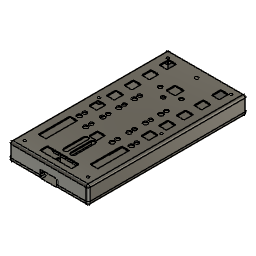
traktorino case v13 (Autodesk Fusion 360 design; units mm, degrees)
Autodesk Fusion 360 part; units mm, degrees
(part 1 of 2)
sketch "Sketch4" plane through (0, 0, 0) normal (0, 0, 1) x (1, 0, 0)
  line L0 (6.0259, 3.0477) -> (114.9323, 3.0477)
  arc A0 (114.9323, 3.0477) -> (119.7795, -1.7995) centre (114.9323, -1.7995) cw
  line L1 (119.7795, -1.7995) -> (119.7795, -228.5675)
  arc A1 (119.7795, -228.5675) -> (114.9323, -233.4147) centre (114.9323, -228.5675) cw
  line L2 (114.9323, -233.4147) -> (6.0259, -233.4147)
  arc A2 (6.0259, -233.4147) -> (1.1787, -228.5675) centre (6.0259, -228.5675) cw
  line L3 (1.1787, -228.5675) -> (1.1787, -1.7995)
  arc A3 (1.1787, -1.7995) -> (6.0259, 3.0477) centre (6.0259, -1.7995) cw
  line L4 (54.6466, -37.8457) -> (66.6101, -37.8457)
  arc A4 (66.6101, -37.8457) -> (67.4219, -38.6575) centre (66.6101, -38.6575) cw
  line L5 (67.4219, -38.6575) -> (67.4219, -51.7349)
  arc A5 (67.4219, -51.7349) -> (66.6101, -52.5468) centre (66.6101, -51.7349) cw
  line L6 (66.6101, -52.5468) -> (54.6466, -52.5468)
  arc A6 (54.6466, -52.5468) -> (53.8348, -51.7349) centre (54.6466, -51.7349) cw
  line L7 (53.8348, -51.7349) -> (53.8348, -38.6575)
  arc A7 (53.8348, -38.6575) -> (54.6466, -37.8457) centre (54.6466, -38.6575) cw
  line L8 (94.2203, -37.1462) -> (104.2753, -37.1462)
  arc A8 (104.2753, -37.1462) -> (105.0525, -37.9233) centre (104.2753, -37.9233) cw
  line L9 (105.0525, -37.9233) -> (105.0525, -50.1841)
  arc A9 (105.0525, -50.1841) -> (104.2753, -50.9613) centre (104.2753, -50.1841) cw
  line L10 (104.2753, -50.9613) -> (94.2203, -50.9613)
  arc A10 (94.2203, -50.9613) -> (93.4431, -50.1841) centre (94.2203, -50.1841) cw
  line L11 (93.4431, -50.1841) -> (93.4431, -37.9233)
  arc A11 (93.4431, -37.9233) -> (94.2203, -37.1462) centre (94.2203, -37.9233) cw
  line L12 (94.2203, -63.1605) -> (104.2753, -63.1605)
  arc A12 (104.2753, -63.1605) -> (105.0525, -63.9377) centre (104.2753, -63.9377) cw
  line L13 (105.0525, -63.9377) -> (105.0525, -76.1984)
  arc A13 (105.0525, -76.1984) -> (104.2753, -76.9756) centre (104.2753, -76.1984) cw
  line L14 (104.2753, -76.9756) -> (94.2203, -76.9756)
  arc A14 (94.2203, -76.9756) -> (93.4431, -76.1984) centre (94.2203, -76.1984) cw
  line L15 (93.4431, -76.1984) -> (93.4431, -63.9377)
  arc A15 (93.4431, -63.9377) -> (94.2203, -63.1605) centre (94.2203, -63.9377) cw
  line L16 (94.2203, -89.1736) -> (104.2753, -89.1736)
  arc A16 (104.2753, -89.1736) -> (105.0525, -89.9507) centre (104.2753, -89.9507) cw
  line L17 (105.0525, -89.9507) -> (105.0525, -102.2115)
  arc A17 (105.0525, -102.2115) -> (104.2753, -102.9887) centre (104.2753, -102.2115) cw
  line L18 (104.2753, -102.9887) -> (94.2203, -102.9887)
  arc A18 (94.2203, -102.9887) -> (93.4431, -102.2115) centre (94.2203, -102.2115) cw
  line L19 (93.4431, -102.2115) -> (93.4431, -89.9507)
  arc A19 (93.4431, -89.9507) -> (94.2203, -89.1736) centre (94.2203, -89.9507) cw
  line L20 (17.1824, -63.1605) -> (27.2374, -63.1605)
  arc A20 (27.2374, -63.1605) -> (28.0146, -63.9377) centre (27.2374, -63.9377) cw
  line L21 (28.0146, -63.9377) -> (28.0146, -76.1984)
  arc A21 (28.0146, -76.1984) -> (27.2374, -76.9756) centre (27.2374, -76.1984) cw
  line L22 (27.2374, -76.9756) -> (17.1824, -76.9756)
  arc A22 (17.1824, -76.9756) -> (16.4052, -76.1984) centre (17.1824, -76.1984) cw
  line L23 (16.4052, -76.1984) -> (16.4052, -63.9377)
  arc A23 (16.4052, -63.9377) -> (17.1824, -63.1605) centre (17.1824, -63.9377) cw
  line L24 (17.1824, -89.1736) -> (27.2374, -89.1736)
  arc A24 (27.2374, -89.1736) -> (28.0146, -89.9507) centre (27.2374, -89.9507) cw
  line L25 (28.0146, -89.9507) -> (28.0146, -102.2115)
  arc A25 (28.0146, -102.2115) -> (27.2374, -102.9887) centre (27.2374, -102.2115) cw
  line L26 (27.2374, -102.9887) -> (17.1824, -102.9887)
  arc A26 (17.1824, -102.9887) -> (16.4052, -102.2115) centre (17.1824, -102.2115) cw
  line L27 (16.4052, -102.2115) -> (16.4052, -89.9507)
  arc A27 (16.4052, -89.9507) -> (17.1824, -89.1736) centre (17.1824, -89.9507) cw
  line L28 (17.1824, -115.1879) -> (27.2374, -115.1879)
  arc A28 (27.2374, -115.1879) -> (28.0146, -115.965) centre (27.2374, -115.965) cw
  line L29 (28.0146, -115.965) -> (28.0146, -128.2258)
  arc A29 (28.0146, -128.2258) -> (27.2374, -129.003) centre (27.2374, -128.2258) cw
  line L30 (27.2374, -129.003) -> (17.1824, -129.003)
  arc A30 (17.1824, -129.003) -> (16.4052, -128.2258) centre (17.1824, -128.2258) cw
  line L31 (16.4052, -128.2258) -> (16.4052, -115.965)
  arc A31 (16.4052, -115.965) -> (17.1824, -115.1879) centre (17.1824, -115.965) cw
  line L32 (94.2203, -115.1879) -> (104.2753, -115.1879)
  arc A32 (104.2753, -115.1879) -> (105.0525, -115.965) centre (104.2753, -115.965) cw
  line L33 (105.0525, -115.965) -> (105.0525, -128.2258)
  arc A33 (105.0525, -128.2258) -> (104.2753, -129.003) centre (104.2753, -128.2258) cw
  line L34 (104.2753, -129.003) -> (94.2203, -129.003)
  arc A34 (94.2203, -129.003) -> (93.4431, -128.2258) centre (94.2203, -128.2258) cw
  line L35 (93.4431, -128.2258) -> (93.4431, -115.965)
  arc A35 (93.4431, -115.965) -> (94.2203, -115.1879) centre (94.2203, -115.965) cw
  line L36 (55.9504, -154.9584) -> (66.0054, -154.9584)
  arc A36 (66.0054, -154.9584) -> (66.7826, -155.7356) centre (66.0054, -155.7356) cw
  line L37 (66.7826, -155.7356) -> (66.7826, -167.9964)
  arc A37 (66.7826, -167.9964) -> (66.0054, -168.7735) centre (66.0054, -167.9964) cw
  line L38 (66.0054, -168.7735) -> (55.9504, -168.7735)
  arc A38 (55.9504, -168.7735) -> (55.1732, -167.9964) centre (55.9504, -167.9964) cw
  line L39 (55.1732, -167.9964) -> (55.1732, -155.7356)
  arc A39 (55.1732, -155.7356) -> (55.9504, -154.9584) centre (55.9504, -155.7356) cw
  line L40 (94.2203, -11.1331) -> (104.2753, -11.1331)
  arc A40 (104.2753, -11.1331) -> (105.0525, -11.9103) centre (104.2753, -11.9103) cw
  line L41 (105.0525, -11.9103) -> (105.0525, -24.1711)
  arc A41 (105.0525, -24.1711) -> (104.2753, -24.9482) centre (104.2753, -24.1711) cw
  line L42 (104.2753, -24.9482) -> (94.2203, -24.9482)
  arc A42 (94.2203, -24.9482) -> (93.4431, -24.1711) centre (94.2203, -24.1711) cw
  line L43 (93.4431, -24.1711) -> (93.4431, -11.9103)
  arc A43 (93.4431, -11.9103) -> (94.2203, -11.1331) centre (94.2203, -11.9103) cw
  line L44 (17.1824, -37.1462) -> (27.2374, -37.1462)
  arc A44 (27.2374, -37.1462) -> (28.0146, -37.9233) centre (27.2374, -37.9233) cw
  line L45 (28.0146, -37.9233) -> (28.0146, -50.1841)
  arc A45 (28.0146, -50.1841) -> (27.2374, -50.9613) centre (27.2374, -50.1841) cw
  line L46 (27.2374, -50.9613) -> (17.1824, -50.9613)
  arc A46 (17.1824, -50.9613) -> (16.4052, -50.1841) centre (17.1824, -50.1841) cw
  line L47 (16.4052, -50.1841) -> (16.4052, -37.9233)
  arc A47 (16.4052, -37.9233) -> (17.1824, -37.1462) centre (17.1824, -37.9233) cw
  line L48 (17.1824, -11.1331) -> (27.2374, -11.1331)
  arc A48 (27.2374, -11.1331) -> (28.0146, -11.9103) centre (27.2374, -11.9103) cw
  line L49 (28.0146, -11.9103) -> (28.0146, -24.1711)
  arc A49 (28.0146, -24.1711) -> (27.2374, -24.9482) centre (27.2374, -24.1711) cw
  line L50 (27.2374, -24.9482) -> (17.1824, -24.9482)
  arc A50 (17.1824, -24.9482) -> (16.4052, -24.1711) centre (17.1824, -24.1711) cw
  line L51 (16.4052, -24.1711) -> (16.4052, -11.9103)
  arc A51 (16.4052, -11.9103) -> (17.1824, -11.1331) centre (17.1824, -11.9103) cw
  line L52 (92.7172, -156.5242) -> (103.2803, -156.5242)
  arc A52 (103.2803, -156.5242) -> (104.1012, -157.345) centre (103.2803, -157.345) cw
  line L53 (104.1012, -157.345) -> (104.1012, -202.6869)
  arc A53 (104.1012, -202.6869) -> (103.2803, -203.5077) centre (103.2803, -202.6869) cw
  line L54 (103.2803, -203.5077) -> (92.7172, -203.5077)
  arc A54 (92.7172, -203.5077) -> (91.8963, -202.6869) centre (92.7172, -202.6869) cw
  line L55 (91.8963, -202.6869) -> (91.8963, -157.345)
  arc A55 (91.8963, -157.345) -> (92.7172, -156.5242) centre (92.7172, -157.345) cw
  line L56 (37.2368, -222.3173) -> (37.2368, -211.7541)
  arc A56 (37.2368, -211.7541) -> (38.0577, -210.9333) centre (38.0577, -211.7541) cw
  line L57 (38.0577, -210.9333) -> (83.3995, -210.9333)
  arc A57 (83.3995, -210.9333) -> (84.2204, -211.7541) centre (83.3995, -211.7541) cw
  line L58 (84.2204, -211.7541) -> (84.2204, -222.3173)
  arc A58 (84.2204, -222.3173) -> (83.3995, -223.1381) centre (83.3995, -222.3173) cw
  line L59 (83.3995, -223.1381) -> (38.0577, -223.1381)
  arc A59 (38.0577, -223.1381) -> (37.2368, -222.3173) centre (38.0577, -222.3173) cw
  line L60 (16.1774, -156.5242) -> (26.7405, -156.5242)
  arc A60 (26.7405, -156.5242) -> (27.5614, -157.345) centre (26.7405, -157.345) cw
  line L61 (27.5614, -157.345) -> (27.5614, -202.6869)
  arc A61 (27.5614, -202.6869) -> (26.7405, -203.5077) centre (26.7405, -202.6869) cw
  line L62 (26.7405, -203.5077) -> (16.1774, -203.5077)
  arc A62 (16.1774, -203.5077) -> (15.3565, -202.6869) centre (16.1774, -202.6869) cw
  line L63 (15.3565, -202.6869) -> (15.3565, -157.345)
  arc A63 (15.3565, -157.345) -> (16.1774, -156.5242) centre (16.1774, -157.345) cw
  circle A64 centre (107.1093, -9.6234) radius 1.5463
  circle A65 centre (13.8605, -9.6234) radius 1.5463
  circle A66 centre (13.8605, -111.1767) radius 1.5463
  circle A67 centre (13.8605, -220.7337) radius 1.5463
  circle A68 centre (107.1093, -220.7337) radius 1.5463
  circle A69 centre (106.1086, -111.1767) radius 1.5463
  circle A70 centre (60.63, -63.4567) radius 4.002
  circle A71 centre (45.122, -52.2009) radius 4.002
  circle A72 centre (76.2883, -52.2009) radius 4.002
  circle A73 centre (41.2196, -78.4647) radius 4.002
  circle A74 centre (80.4403, -78.4647) radius 4.002
  circle A75 centre (80.2404, -101.2262) radius 4.002
  circle A76 centre (41.2196, -101.2262) radius 4.002
  circle A77 centre (41.2196, -125.239) radius 4.002
  circle A78 centre (80.2404, -125.239) radius 4.002
  circle A79 centre (41.2196, -150.2522) radius 4.002
  circle A80 centre (80.2404, -150.2522) radius 4.002
  circle A81 centre (22.4601, -140.747) radius 4.002
  circle A82 centre (99.1501, -140.697) radius 4.002
  circle A83 centre (60.4541, -13.652) radius 2.5179
  line L64 (55.546, -169.3438) -> (56.0576, -169.3438)
  arc A84 (56.0576, -169.3438) -> (59.1753, -172.4614) centre (56.0576, -172.4614) cw
  line L65 (59.1753, -172.4614) -> (59.1753, -202.0242)
  arc A85 (59.1753, -202.0242) -> (56.0576, -205.1418) centre (56.0576, -202.0242) cw
  line L66 (56.0576, -205.1418) -> (55.546, -205.1418)
  arc A86 (55.546, -205.1418) -> (52.4283, -202.0242) centre (55.546, -202.0242) cw
  line L67 (52.4283, -202.0242) -> (52.4283, -172.4614)
  arc A87 (52.4283, -172.4614) -> (55.546, -169.3438) centre (55.546, -172.4614) cw
  line L68 (65.903, -169.3438) -> (66.4147, -169.3438)
  arc A88 (66.4147, -169.3438) -> (69.5323, -172.4614) centre (66.4147, -172.4614) cw
  line L69 (69.5323, -172.4614) -> (69.5323, -202.0242)
  arc A89 (69.5323, -202.0242) -> (66.4147, -205.1418) centre (66.4147, -202.0242) cw
  line L70 (66.4147, -205.1418) -> (65.903, -205.1418)
  arc A90 (65.903, -205.1418) -> (62.7854, -202.0242) centre (65.903, -202.0242) cw
  line L71 (62.7854, -202.0242) -> (62.7854, -172.4614)
  arc A91 (62.7854, -172.4614) -> (65.903, -169.3438) centre (65.903, -172.4614) cw
  circle A92 centre (41.2196, -86.5647) radius 3.5
  circle A93 centre (41.2196, -109.3262) radius 3.5
  circle A94 centre (41.2196, -133.339) radius 3.5
  circle A95 centre (41.2196, -158.3522) radius 3.5
  circle A96 centre (22.4601, -148.847) radius 3.5
  circle A97 centre (80.4403, -158.3522) radius 3.5
  circle A98 centre (99.1501, -148.797) radius 3.5
  circle A99 centre (80.4403, -109.3262) radius 3.5
  circle A100 centre (80.4403, -86.5647) radius 3.5
  line L72 (60.4791, 3.0477) -> (60.4791, -233.4147) construction
  line L73 (99.1501, -140.697) -> (99.1501, -156.5242) construction
  line L74 (22.4601, -140.747) -> (22.4601, -156.5242) construction
  line L75 (76.2883, -52.2009) -> (76.2883, -233.4147) construction
  line L76 (45.122, -52.2009) -> (45.122, -233.4147) construction
  line L77 (41.2196, -78.4647) -> (41.2196, -233.4147) construction
  line L78 (80.4403, -78.4647) -> (80.4403, -233.4147) construction
  circle A101 centre (80.4403, -133.339) radius 3.5
  line L79 (66.4147, -206.1418) -> (65.903, -206.1418)
  line L80 (56.0576, -205.5193) -> (55.546, -205.5193)
  line L81 (91.8963, -201.6869) -> (91.8963, -156.345)
  arc A102 (91.8963, -156.345) -> (92.7172, -155.5242) centre (92.7172, -156.345) cw
  line L82 (92.7172, -155.5242) -> (103.2803, -155.5242)
  arc A103 (103.2803, -155.5242) -> (104.1012, -156.345) centre (103.2803, -156.345) cw
  line L83 (104.1012, -156.345) -> (104.1012, -201.6869)
  line L84 (16.1774, -155.5242) -> (26.7405, -155.5242)
  arc A104 (15.3565, -156.345) -> (16.1774, -155.5242) centre (16.1774, -156.345) cw
  line L85 (15.3565, -201.6869) -> (15.3565, -156.345)
  arc A105 (26.7405, -155.5242) -> (27.5614, -156.345) centre (26.7405, -156.345) cw
  line L86 (27.5614, -156.345) -> (27.5614, -201.6869)
  circle A106 centre (107.1093, -9.6234) radius 1.85
  circle A107 centre (13.8605, -9.6234) radius 1.85
  circle A108 centre (13.8605, -220.7337) radius 1.85
  circle A109 centre (107.1093, -220.7337) radius 1.85
  circle A110 centre (106.1086, -111.1767) radius 1.85
  circle A111 centre (13.8605, -111.1767) radius 1.85
  line L87 (33.4146, -9.7764) -> (32.2146, -9.7764)
  line L88 (32.2146, -9.7764) -> (32.2146, -170.7764)
  line L89 (32.2146, -170.7764) -> (33.4146, -170.7764)
  line L90 (33.4146, -170.7764) -> (33.4146, -9.7764)
  line L91 (88.7437, -9.7764) -> (88.7437, -170.7764)
  line L92 (87.5437, -170.7764) -> (87.5437, -9.7764)
  line L93 (87.5437, -9.7764) -> (88.7437, -9.7764)
  line L94 (88.7437, -170.7764) -> (87.5437, -170.7764)
  line L95 (61.4753, -170.0735) -> (60.2753, -170.0735)
  line L96 (60.2753, -170.0735) -> (60.2753, -208.9333)
  line L97 (60.2753, -208.9333) -> (61.4753, -208.9333)
  line L98 (61.4753, -208.9333) -> (61.4753, -170.0735)
  line L99 (77.9548, -207.7333) -> (42.9548, -207.7333)
  line L100 (42.9548, -207.7333) -> (42.9548, -208.9333)
  line L101 (42.9548, -208.9333) -> (77.9548, -208.9333)
  line L102 (77.9548, -208.9333) -> (77.9548, -207.7333)
  line L103 (9.4791, -225.1835) -> (111.4791, -225.1835)
  line L104 (111.4791, -225.1835) -> (111.4791, -5.1835)
  line L105 (111.4791, -5.1835) -> (9.4791, -5.1835)
  line L106 (9.4791, -5.1835) -> (9.4791, -225.1835)
  line L107 (111.4791, -115.1835) -> (9.4791, -115.1835) construction
  line L108 (113.0791, -226.7835) -> (113.0791, -3.5835)
  line L109 (113.0791, -3.5835) -> (7.8791, -3.5835)
  line L110 (7.8791, -3.5835) -> (7.8791, -226.7835)
  line L111 (7.8791, -226.7835) -> (113.0791, -226.7835)
  line L112 (4.4791, -0.1835) -> (4.4791, -230.1835)
  line L113 (4.4791, -230.1835) -> (116.4791, -230.1835)
  line L114 (116.4791, -230.1835) -> (116.4791, -0.1835)
  line L115 (116.4791, -0.1835) -> (4.4791, -0.1835)
  line L116 (2.0791, 2.2165) -> (2.0791, -232.5835)
  line L117 (2.0791, -232.5835) -> (118.8791, -232.5835)
  line L118 (118.8791, -232.5835) -> (118.8791, 2.2165)
  line L119 (118.8791, 2.2165) -> (2.0791, 2.2165)
  line L120 (113.0791, -3.5835) -> (118.8791, -6.9321)
  line L121 (113.0791, -3.5835) -> (118.0217, -3.5835) construction
  line L122 (113.0791, -226.7835) -> (113.0791, -222.1876)
  line L123 (113.0791, -226.7835) -> (118.8791, -223.4349)
  line L124 (113.0791, -226.7835) -> (118.0217, -226.7835) construction
  line L125 (7.8791, -226.7835) -> (2.0791, -223.4349)
  line L126 (7.8791, -3.5835) -> (2.0791, -6.9321)
  line L127 (111.4791, -225.1835) -> (105.2593, -225.1835)
  line L128 (105.2593, -225.1835) -> (105.2593, -218.8837)
  line L129 (105.2593, -218.8837) -> (111.4791, -218.8837)
  line L130 (111.4791, -218.8837) -> (111.4791, -225.1835)
  line L131 (9.4791, -225.1835) -> (15.7105, -225.1835)
  line L132 (15.7105, -225.1835) -> (15.7105, -218.8837)
  line L133 (15.7105, -218.8837) -> (9.4791, -218.8837)
  line L134 (9.4791, -218.8837) -> (9.4791, -225.1835)
  line L135 (111.4791, -5.1835) -> (105.2593, -5.1835)
  line L136 (105.2593, -5.1835) -> (105.2593, -11.4734)
  line L137 (105.2593, -11.4734) -> (111.4791, -11.4734)
  line L138 (111.4791, -11.4734) -> (111.4791, -5.1835)
  line L139 (9.4791, -5.1835) -> (15.7105, -5.1835)
  line L140 (15.7105, -5.1835) -> (15.7105, -11.4734)
  line L141 (15.7105, -11.4734) -> (9.4791, -11.4734)
  line L142 (9.4791, -11.4734) -> (9.4791, -5.1835)
  line L143 (111.4791, -225.1835) -> (104.2593, -225.1835)
  line L144 (104.2593, -225.1835) -> (104.2593, -217.8837)
  line L145 (104.2593, -217.8837) -> (111.4791, -217.8837)
  line L146 (111.4791, -217.8837) -> (111.4791, -225.1835)
  line L147 (16.6989, -225.1835) -> (16.6989, -217.8837)
  line L148 (16.6989, -217.8837) -> (9.4791, -217.8837)
  line L149 (104.2593, -12.4833) -> (111.4791, -12.4833)
  line L150 (104.2593, -5.1835) -> (104.2593, -12.4833)
  line L151 (16.6989, -12.4833) -> (9.4791, -12.4833)
  line L152 (16.6989, -5.1835) -> (16.6989, -12.4833)
  line L153 (9.4791, -114.0267) -> (111.4791, -114.0267)
  line L154 (111.4791, -108.3267) -> (9.4791, -108.3267)
  line L155 (16.7105, -114.0267) -> (16.7105, -108.3267)
  line L156 (103.2586, -114.0267) -> (103.2586, -108.3267)
  line L157 (53.8348, -52.9349) -> (53.8348, -39.8575)
  arc A112 (53.8348, -39.8575) -> (54.6466, -39.0457) centre (54.6466, -39.8575) cw
  line L158 (54.6466, -39.0457) -> (66.6101, -39.0457)
  arc A113 (66.6101, -39.0457) -> (67.4219, -39.8575) centre (66.6101, -39.8575) cw
  line L159 (67.4219, -39.8575) -> (67.4219, -52.9349)
  circle A114 centre (45.122, -52.2009) radius 3.002
  circle A115 centre (60.63, -63.4567) radius 3.002
  circle A116 centre (76.2883, -52.2009) radius 3.002
  circle A117 centre (41.2196, -78.4647) radius 3.002
  circle A118 centre (80.4403, -78.4647) radius 3.002
  circle A119 centre (41.2196, -101.2262) radius 3.002
  circle A120 centre (80.2404, -101.2262) radius 3.002
  circle A121 centre (80.2404, -125.239) radius 3.002
  circle A122 centre (41.2196, -125.239) radius 3.002
  circle A123 centre (22.4601, -140.747) radius 3.002
  circle A124 centre (41.2196, -150.2522) radius 3.002
  circle A125 centre (99.1501, -140.697) radius 3.002
  circle A126 centre (80.2404, -150.2522) radius 3.002
  line L160 (92.3963, -202.6869) -> (92.3963, -157.345)
  arc A127 (92.7172, -157.0242) -> (92.3963, -157.345) centre (92.7172, -157.345) ccw
  line L161 (92.7172, -157.0242) -> (103.2803, -157.0242)
  arc A128 (103.6012, -157.345) -> (103.2803, -157.0242) centre (103.2803, -157.345) ccw
  line L162 (103.6012, -157.345) -> (103.6012, -202.6869)
  arc A129 (103.2803, -203.0077) -> (103.6012, -202.6869) centre (103.2803, -202.6869) ccw
  line L163 (103.2803, -203.0077) -> (92.7172, -203.0077)
  arc A130 (92.3963, -202.6869) -> (92.7172, -203.0077) centre (92.7172, -202.6869) ccw
  line L164 (92.3963, -202.0869) -> (92.3963, -156.745)
  arc A131 (92.7172, -156.4242) -> (92.3963, -156.745) centre (92.7172, -156.745) ccw
  line L165 (92.7172, -156.4242) -> (103.2803, -156.4242)
  arc A132 (103.6012, -156.745) -> (103.2803, -156.4242) centre (103.2803, -156.745) ccw
  line L166 (103.6012, -156.745) -> (103.6012, -202.0869)
  line L167 (55.1732, -166.9964) -> (55.1732, -154.7356)
  arc A133 (55.9504, -167.7735) -> (55.1732, -166.9964) centre (55.9504, -166.9964) cw
  line L168 (66.0054, -167.7735) -> (55.9504, -167.7735)
  arc A134 (66.7826, -166.9964) -> (66.0054, -167.7735) centre (66.0054, -166.9964) cw
  line L169 (66.7826, -154.7356) -> (66.7826, -166.9964)
  line L170 (26.7405, -203.0077) -> (16.1774, -203.0077)
  arc A135 (15.8565, -202.6869) -> (16.1774, -203.0077) centre (16.1774, -202.6869) ccw
  line L171 (15.8565, -202.6869) -> (15.8565, -157.345)
  arc A136 (16.1774, -157.0242) -> (15.8565, -157.345) centre (16.1774, -157.345) ccw
  line L172 (16.1774, -157.0242) -> (26.7405, -157.0242)
  arc A137 (27.0614, -157.345) -> (26.7405, -157.0242) centre (26.7405, -157.345) ccw
  line L173 (27.0614, -157.345) -> (27.0614, -202.6869)
  arc A138 (26.7405, -203.0077) -> (27.0614, -202.6869) centre (26.7405, -202.6869) ccw
  line L174 (15.8565, -202.0869) -> (15.8565, -156.745)
  line L175 (16.1774, -156.4242) -> (26.7405, -156.4242)
  arc A139 (16.1774, -156.4242) -> (15.8565, -156.745) centre (16.1774, -156.745) ccw
  line L176 (27.0614, -156.745) -> (27.0614, -202.0869)
  arc A140 (27.0614, -156.745) -> (26.7405, -156.4242) centre (26.7405, -156.745) ccw
  line L177 (37.2368, -221.3173) -> (37.2368, -210.7541)
  arc A141 (38.0577, -222.1381) -> (37.2368, -221.3173) centre (38.0577, -221.3173) cw
  line L178 (83.3995, -222.1381) -> (38.0577, -222.1381)
  arc A142 (84.2204, -221.3173) -> (83.3995, -222.1381) centre (83.3995, -221.3173) cw
  line L179 (84.2204, -210.7541) -> (84.2204, -221.3173)
  point P0 (108.6555, -9.6234)
  point P1 (15.4068, -9.6234)
  point P2 (15.4068, -111.1767)
  point P3 (15.4068, -220.7337)
  point P4 (108.6555, -220.7337)
  point P5 (107.6548, -111.1767)
  point P6 (64.6321, -63.4567)
  point P7 (49.124, -52.2009)
  point P8 (80.2903, -52.2009)
  point P9 (45.2217, -78.4647)
  point P10 (84.4423, -78.4647)
  point P11 (84.2424, -101.2262)
  point P12 (45.2217, -101.2262)
  point P13 (45.2217, -125.239)
  point P14 (84.2424, -125.239)
  point P15 (45.2217, -150.2522)
  point P16 (84.2424, -150.2522)
  point P17 (26.5202, -140.747)
  point P18 (103.1521, -140.697)
  point P19 (62.972, -13.652)
  point P20 (60.4791, -115.1835)
  point P21 (60.4791, -115.1835)
  dimension "d28" = 8.1
  dimension "d29" = 8.1
  dimension "d30" = 8.1
  dimension "d31" = 8.1
  dimension "d35" = 8.1
  dimension "d36" = 8.1
  dimension "d37" = 8.1
  dimension "d38" = 8.1
  dimension "d39" = 8.1
  dimension "d40" = 8.1
  dimension "d44" = 7
  dimension "d45" = 7
  dimension "d46" = 7
  dimension "d47" = 7
  dimension "d48" = 7
  dimension "d49" = 7
  dimension "d50" = 7
  dimension "d51" = 7
  dimension "d52" = 7
  dimension "d53" = 7
  dimension "d56" = 3.7
  dimension "d58" = 3.7
  dimension "d59" = 3.7
  dimension "d60" = 3.7
  dimension "d61" = 3.7
  dimension "d62" = 3.7
  dimension "d64" = 1.2
  dimension "d65" = 161
  dimension "d66" = 4.2
  dimension "d67" = 1.2
  dimension "d69" = 1.3
  dimension "d70" = 2
  dimension "d71" = 35
  dimension "d72" = 1.2
  dimension "d73" = 2
  dimension "d79" = 102
  dimension "d80" = 220
  dimension "d81" = 1.6
  dimension "d89" = 5
  dimension "d93" = 7.4
  dimension "d94" = 30
  dimension "d95" = 120
  dimension "d96" = 30
  dimension "d110" = 1
  dimension "d111" = 1
  dimension "d112" = 2.85
  dimension "d113" = 2.85
  dimension "d114" = 2.85
  dimension "d115" = 2.85
  dimension "d221" = 1
  dimension "d222" = 1
  dimension "d223" = 1
  dimension "d224" = 1
  dimension "d225" = 1
  dimension "d226" = 1
  dimension "d227" = 1
  dimension "d228" = 1
  dimension "d229" = 1
  dimension "d230" = 1
  dimension "d231" = 1
  dimension "d232" = 1
  dimension "d233" = 1
  dimension "d234" = 0.5
  dimension "d235" = 0.5
  constraint midpoint L0 L72.start
  constraint midpoint L2 L72.end
  constraint coincident A82.centre L73.start
  constraint coincident L52 L73.end
  constraint perpendicular L52 L73
  constraint coincident A81.centre L74.start
  constraint coincident L60 L74.end
  constraint perpendicular L60 L74
  constraint coincident A72.centre L75.start
  constraint coincident L2 L75.end
  constraint perpendicular L2 L75
  constraint coincident A71.centre L76.start
  constraint coincident L2 L76.end
  constraint perpendicular L2 L76
  constraint coincident A73.centre L77.start
  constraint coincident L2 L77.end
  constraint perpendicular L2 L77
  constraint coincident A74.centre L78.start
  constraint coincident L2 L78.end
  constraint perpendicular L2 L78
  constraint coincident A97.centre L78
  constraint coincident A98.centre L73
  constraint coincident A99.centre L78
  constraint coincident A100.centre L78
  constraint coincident A96.centre L74
  constraint coincident A95.centre L77
  constraint coincident A94.centre L77
  constraint coincident A93.centre L77
  constraint coincident A92.centre L77
  constraint coincident L78 A101.centre
  constraint concentric A64 A106
  constraint concentric A65 A107
  constraint concentric A67 A108
  constraint concentric A68 A109
  constraint concentric A69 A110
  constraint concentric A66 A111
  constraint horizontal L87
  constraint vertical L88
  constraint horizontal L89
  constraint vertical L90
  constraint symmetric L72 L87.start L92.end
  constraint symmetric L72 L87.end L91.start
  constraint symmetric L72 L88.end L91.end
  constraint symmetric L72 L89.end L92.start
  constraint horizontal L95
  constraint vertical L96
  constraint horizontal L97
  constraint vertical L98
  constraint horizontal L99
  constraint vertical L100
  constraint horizontal L101
  constraint vertical L102
  constraint midpoint L72 P21
  constraint horizontal L103
  constraint vertical L104
  constraint horizontal L105
  constraint vertical L106
  constraint midpoint L104 L107.start
  constraint midpoint L106 L107.end
  constraint midpoint L107 P21
  constraint coincident P21 P20
  constraint horizontal L121
  constraint coincident L118 L120.end
  constraint horizontal L124
  constraint coincident L118 L123.end
  constraint symmetric L72 L108.start L110.end
  constraint symmetric L72 L108.end L109.end
  constraint symmetric L72 L120.end L126.end
  constraint symmetric L72 L123.end L125.end
  constraint horizontal L127
  constraint vertical L128
  constraint horizontal L129
  constraint vertical L130
  constraint tangent A109 L129
  constraint tangent A109 L128
  constraint horizontal L131
  constraint vertical L132
  constraint horizontal L133
  constraint vertical L134
  constraint tangent A108 L132
  constraint tangent A108 L133
  constraint horizontal L135
  constraint vertical L136
  constraint horizontal L137
  constraint vertical L138
  constraint tangent A106 L137
  constraint tangent A106 L136
  constraint horizontal L139
  constraint vertical L140
  constraint horizontal L141
  constraint vertical L142
  constraint tangent A107 L141
  constraint tangent A107 L140
  constraint horizontal L143
  constraint vertical L144
  constraint horizontal L145
  constraint vertical L146
  constraint symmetric L72 L143.end L147.start
  constraint symmetric L72 L144.end L147.end
  constraint symmetric L72 L145.end L148.end
  constraint symmetric L107 L143.end L150.start
  constraint symmetric L107 L144.end L149.start
  constraint symmetric L107 L145.end L149.end
  constraint symmetric L107 L147.start L152.start
  constraint symmetric L107 L147.end L151.start
  constraint symmetric L107 L148.end L151.end
  constraint coincident L106 L153.start
  constraint coincident L104 L153.end
  constraint perpendicular L104 L153
  constraint coincident L104 L154.start
  constraint coincident L106 L154.end
  constraint perpendicular L106 L154
  constraint coincident L153 L155.start
  constraint coincident L154 L155.end
  constraint perpendicular L154 L155
  constraint coincident L153 L156.start
  constraint coincident L154 L156.end
  constraint perpendicular L154 L156
  measures "d28" vertical distance of A75.centre A99.centre
  measures "d29" vertical distance of A80.centre A97.centre
  measures "d30" distance of A98.centre A82.centre
  measures "d31" distance of A100.centre A74.centre
  measures "d35" distance of A92.centre A73.centre
  measures "d36" distance of A76.centre A93.centre
  measures "d37" distance of A77.centre A94.centre
  measures "d38" distance of A96.centre A81.centre
  measures "d39" distance of A79.centre A95.centre
  measures "d40" vertical distance of A78.centre A101.centre
  measures "d44" diameter of A97
  measures "d45" diameter of A95
  measures "d46" diameter of A96
  measures "d47" diameter of A98
  measures "d48" diameter of A101
  measures "d49" diameter of A94
  measures "d50" diameter of A93
  measures "d51" diameter of A99
  measures "d52" diameter of A100
  measures "d53" diameter of A92
  measures "d56" diameter of A106
  measures "d58" diameter of A107
  measures "d59" diameter of A108
  measures "d60" diameter of A109
  measures "d61" diameter of A110
  measures "d62" diameter of A111
  measures "d64" distance of L88 L90
  measures "d65" distance of L87 L89
  measures "d66" distance of L49 L88
  measures "d67" distance of L95.start L95.end
  measures "d69" distance of L38 L95
  measures "d70" distance of L57 L97
  measures "d71" distance of L99.start L99.end
  measures "d72" distance of L99.start L101.end
  measures "d73" distance of L57 L101
  measures "d79" distance of L103.start L103.end
  measures "d80" distance of L103.start L105.end
  measures "d94" angle of L120 L121
  measures "d95" angle of L120 L122
  measures "d96" angle of L123 L124
  measures "d110" distance of L129 L145
  measures "d111" distance of L128 L144
  measures "d112" distance of A66.centre L154
  measures "d113" distance of A66.centre L153
  measures "d114" distance of A66.centre L155
  measures "d115" distance of A69.centre L156
extrude "Extrude4" add sketch "Sketch4" along normal blind 1.6 contours A0 A3 L112 L114 L115 L116 L118 L119 L120 L126 | A3 L116 L119 | A0 L118 L119 | L112 L116 L125 L126 | L114 L118 L120 L123 | A1 A2 L112 L113 L114 L116 L117 L118 L123 L125 | L110 L112 L125 L126 | L109 L112 L114 L115 L120 L126 | L108 L114 L120 L122 L123 | A2 L116 L117 | L111 L112 L113 L114 L123 L125 | L108 L109 L110 L111 L122 | A1 L117 L118 | L4 A4 L5 L7 A7 A112 L158 A113 | L37 A37 L38 A38 L39 A133 L168 A134 | L40 L41 A41 L42 A42 L43 A43 L48 A48 L49 A49 L50 A50 L51 A51 A93 A99 L87 L88 L90 L91 L92 L93 L104 L105 L106 L149 L150 L151 L152 L154 | L40 A40 L41 L104 L105 L136 L137 L149 L150 | A106 L104 L105 L135 L136 L137 L138 | L51 A51 L105 L106 L140 L141 L151 L152 | A106 L136 L137 | A107 L105 L106 L139 L140 L141 L142 | A107 L140 L141 | L104 L153 L154 L156 | L88 L89 L90 L91 L92 L94 L103 L104 L106 L144 L145 L147 L148 L153 | L91 L153 L154 L156 | L103 L104 L128 L129 L143 L144 L145 L146 | L91 L92 L93 L154 | L91 L92 L153 L154 | L106 L153 L154 L155 | A109 L103 L104 L127 L128 L129 L130 L143 L146 | L91 L92 L94 L153 | A93 A99 L90 L92 L153 L154 | L88 L153 L154 L155 | A109 L128 L129 | L103 L106 L132 L133 L147 L148 | L88 L90 L153 L154 | L87 L88 L90 L154 | L88 L89 L90 L153 | A108 L103 L106 L131 L132 L133 L134 | A108 L132 L133 | A52 L53 A53 L54 A54 L55 A55 L81 L83 L160 L162 A129 L163 A130 L164 A131 A132 L166 | A52 A55 L81 A102 L82 A103 L83 A131 L165 A132 | L56 L58 A58 L59 A59 A141 L178 A142 | A60 L61 A61 L62 A62 L63 A63 L85 L86 L170 A135 L171 L173 A138 L174 A139 L176 A140 | A60 A63 L84 A104 L85 A105 L86 L175 A139 A140 | A70 | A71 | A72 | A73 | A74 | A75 | A76 | A77 | A78 | A79 | A80 | A81 | A82 | L95 L96 L98 L99 | L98 L99 L101 L102 | L96 L97 L98 L99 L101 | L96 L99 L100 L101 makes body 1
extrude "Extrude27" add sketch "Sketch4" against normal blind 0.2 from surface at 1.6 contours A83 bodies 1
extrude "Extrude5" add sketch "Sketch4" against normal blind 4.4 contours L40 A40 L41 L104 L105 L136 L137 L149 L150 | A106 L104 L105 L135 L136 L137 L138 | L51 A51 L105 L106 L140 L141 L151 L152 | A106 L136 L137 | A107 L105 L106 L139 L140 L141 L142 | A107 L140 L141 | L104 L153 L154 L156 | L103 L104 L128 L129 L143 L144 L145 L146 | L91 L92 L93 L154 | L91 L92 L153 L154 | L106 L153 L154 L155 | A109 L103 L104 L127 L128 L129 L130 L143 L146 | L91 L92 L94 L153 | A109 L128 L129 | L103 L106 L132 L133 L147 L148 | L88 L90 L153 L154 | L87 L88 L90 L154 | L88 L89 L90 L153 | A108 L103 L106 L131 L132 L133 L134 | A108 L132 L133 | L95 L96 L98 L99 | L98 L99 L101 L102 | L96 L97 L98 L99 L101 | L96 L99 L100 L101 bodies 1
extrude "Extrude7" add sketch "Sketch4" against normal blind 6.2 contours L112 L116 L125 L126 | L114 L118 L120 L123 | L110 L112 L125 L126 | L108 L114 L120 L122 L123 bodies 1
extrude "Extrude6" add sketch "Sketch4" against normal blind 19.2 contours A0 A3 L112 L114 L115 L116 L118 L119 L120 L126 | A3 L116 L119 | A0 L118 L119 | L112 L116 L125 L126 | L114 L118 L120 L123 | A1 A2 L112 L113 L114 L116 L117 L118 L123 L125 | L109 L112 L114 L115 L120 L126 | A2 L116 L117 | L111 L112 L113 L114 L123 L125 | L108 L109 L110 L111 L122 | A1 L117 L118 bodies 1
sketch "Sketch5" plane through (0, 0, -6.2) normal (0, 0, -1) x (1, 0, 0)
  line L0 (116.4791, 5.5465) -> (116.4791, 224.8205)
  line L1 (116.4791, 224.8205) -> (113.0791, 226.7835)
  line L2 (113.0791, 226.7835) -> (113.0791, 3.5835)
  line L3 (113.0791, 3.5835) -> (116.4791, 5.5465)
  circle A0 centre (113.0791, 4.5835) radius 3.4
  line L4 (116.4791, 5.5465) -> (116.4791, 4.5835)
  line L5 (113.0791, 1.1835) -> (98.0791, 1.1835)
  line L6 (98.0791, 1.1835) -> (98.0791, 4.5835)
  line L7 (98.0791, 4.5835) -> (113.0791, 4.5835)
  line L8 (113.0791, 4.5835) -> (113.0791, 1.1835)
  line L9 (113.0791, 4.5835) -> (116.4791, 4.5835)
  line L10 (116.4791, 4.5835) -> (116.4791, 7.9835)
  line L11 (116.4791, 7.9835) -> (113.0791, 7.9835)
  line L12 (113.0791, 7.9835) -> (113.0791, 4.5835)
  line L13 (60.4791, -3.0477) -> (60.4791, 233.4147)
  line L14 (7.8791, 7.9835) -> (7.8791, 4.5835)
  line L15 (22.8791, 4.5835) -> (7.8791, 4.5835)
  line L16 (4.4791, 7.9835) -> (7.8791, 7.9835)
  line L17 (7.8791, 4.5835) -> (7.8791, 1.1835)
  line L18 (4.4791, 5.5465) -> (4.4791, 4.5835)
  line L19 (7.8791, 3.5835) -> (4.4791, 5.5465)
  line L20 (7.8791, 4.5835) -> (4.4791, 4.5835)
  line L21 (7.8791, 1.1835) -> (22.8791, 1.1835)
  circle A1 centre (7.8791, 4.5835) radius 3.4
  line L22 (22.8791, 1.1835) -> (22.8791, 4.5835)
  line L23 (4.4791, 4.5835) -> (4.4791, 7.9835)
  line L24 (98.0791, 4.5835) -> (101.4791, 1.1835)
  line L25 (98.0791, 4.5835) -> (102.2874, 4.5835) construction
  line L26 (22.8791, 4.5835) -> (19.4791, 1.1835)
  line L27 (22.8791, 4.5835) -> (28.2874, 4.5835) construction
  line L28 (111.4791, 115.1835) -> (9.4791, 115.1835)
  circle A2 centre (113.0791, 225.7835) radius 3.4
  line L29 (113.0791, 229.1835) -> (98.0791, 229.1835)
  line L30 (98.0791, 225.7835) -> (101.4791, 229.1835)
  line L31 (113.0791, 225.7835) -> (113.0791, 229.1835)
  line L32 (116.4791, 225.7835) -> (116.4791, 222.3835)
  line L33 (113.0791, 222.3835) -> (113.0791, 225.7835)
  line L34 (98.0791, 225.7835) -> (102.2874, 225.7835) construction
  line L35 (7.8791, 225.7835) -> (4.4791, 225.7835)
  line L36 (4.4791, 224.8205) -> (4.4791, 225.7835)
  line L37 (22.8791, 229.1835) -> (22.8791, 225.7835)
  line L38 (4.4791, 225.7835) -> (4.4791, 222.3835)
  line L39 (7.8791, 226.7835) -> (4.4791, 224.8205)
  line L40 (7.8791, 222.3835) -> (7.8791, 225.7835)
  line L41 (22.8791, 225.7835) -> (28.2874, 225.7835) construction
  line L42 (22.8791, 225.7835) -> (7.8791, 225.7835)
  circle A3 centre (7.8791, 225.7835) radius 3.4
  line L43 (7.8791, 229.1835) -> (22.8791, 229.1835)
  line L44 (4.4791, 222.3835) -> (7.8791, 222.3835)
  line L45 (113.0791, 226.7835) -> (116.4791, 224.8205)
  line L46 (7.8791, 225.7835) -> (7.8791, 229.1835)
  line L47 (116.4791, 224.8205) -> (116.4791, 225.7835)
  line L48 (116.4791, 222.3835) -> (113.0791, 222.3835)
  line L49 (98.0791, 229.1835) -> (98.0791, 225.7835)
  line L50 (113.0791, 225.7835) -> (116.4791, 225.7835)
  line L51 (22.8791, 225.7835) -> (19.4791, 229.1835)
  line L52 (98.0791, 225.7835) -> (113.0791, 225.7835)
  line L53 (98.0791, 225.7835) -> (116.4791, 225.7835)
  line L54 (116.4791, 225.7835) -> (116.4791, 219.1835)
  line L55 (116.4791, 219.1835) -> (98.0791, 219.1835)
  line L56 (98.0791, 219.1835) -> (98.0791, 225.7835)
  line L57 (22.8791, 219.1835) -> (22.8791, 225.7835)
  line L58 (4.4791, 219.1835) -> (22.8791, 219.1835)
  line L59 (4.4791, 225.7835) -> (4.4791, 219.1835)
  point P0 (60.4791, 233.4147)
  point P1 (0, 230.367)
  dimension "d99" = 6.8
  dimension "d100" = 1
  dimension "d101" = 15
  dimension "d102" = 3.4
  dimension "d105" = 3.4
  dimension "d106" = 3.4
  dimension "d107" = 45
  dimension "d108" = 135
  dimension "d180" = 6.6
  constraint coincident L2 A0.centre
  constraint coincident L0.start L3.end
  constraint coincident A0 L4.end
  constraint tangent A0 L4
  constraint horizontal L5
  constraint vertical L6
  constraint horizontal L7
  constraint vertical L8
  constraint coincident A0 L5.start
  constraint coincident L2.end L8
  constraint horizontal L9
  constraint vertical L10
  constraint horizontal L11
  constraint vertical L12
  constraint coincident A0.centre L7.end
  constraint symmetric L0.start L13 L18.start
  constraint symmetric L2.end L13 L19.start
  constraint symmetric A0 L13 A1
  constraint symmetric L4.end L13 L18.end
  constraint symmetric L5.start L13 L17.end
  constraint symmetric L5.end L13 L21.end
  constraint symmetric L6.end L13 L15.start
  constraint symmetric A0.centre L13 L14.end
  constraint symmetric L10.end L13 L16.start
  constraint symmetric L11.end L13 L14.start
  constraint horizontal L25
  constraint coincident L5 L24.end
  constraint horizontal L27
  constraint coincident L21 L26.end
  constraint symmetric origin L28 P1
  constraint symmetric L0.start L28 L0.end
  constraint symmetric L2.end L28 L1.end
  constraint symmetric A0 L28 A2
  constraint symmetric L4.end L28 L32.start
  constraint symmetric L5.start L28 L29.start
  constraint symmetric L5.end L28 L29.end
  constraint symmetric L6.end L28 L30.start
  constraint symmetric A0.centre L28 A2.centre
  constraint symmetric L10.end L28 L32.end
  constraint symmetric L11.end L28 L33.start
  constraint symmetric L13.start L28 P0
  constraint symmetric L15.start L28 L37.end
  constraint symmetric L14.end L28 L35.start
  constraint symmetric L21.end L28 L37.start
  constraint symmetric L14.start L28 L40.start
  constraint symmetric L16.start L28 L38.end
  constraint symmetric L18.end L28 L35.end
  constraint symmetric L19.start L28 L39.start
  constraint symmetric L17.end L28 L43.start
  constraint symmetric L18.start L28 L36.start
  constraint symmetric A1 L28 A3
  constraint symmetric L24.end L28 L30.end
  constraint symmetric L25.end L28 L34.end
  constraint symmetric L26.end L28 L51.end
  constraint symmetric L27.end L28 L41.end
  constraint horizontal L53
  constraint vertical L54
  constraint horizontal L55
  constraint vertical L56
  constraint coincident L0 L54.end
  constraint symmetric L13 L30.start L37.end
  constraint symmetric L13 L32.start L35.end
  constraint symmetric L13 L54.end L58.start
  constraint symmetric L13 L55.end L57.start
  measures "d99" diameter of A0
  measures "d100" distance of L2.end A0.centre
  measures "d101" distance of L5.start L5.end
  measures "d102" distance of L5.start A0.centre
  measures "d105" distance of A0.centre L4.end
  measures "d106" distance of A0.centre L11.end
  measures "d107" angle of L24 L25
  measures "d108" angle of L26 L27
  measures "d180" distance of L53 L55
extrude "Extrude8" cut sketch "Sketch5" along normal blind 13 contours L0 L2 L48 L54 L55 | L0 L1 A2 L32 L45 L48 L54 | L2 A2 L52 L53 L55 L56 | L1 A2 L32 L45 L47 L54 | L2 A2 L33 L52 L53 | L1 L2 A2 L33 L45 L50 L53 | L1 A2 L45 L50 L53 | L1 A2 L31 L45 L50 L53 | L2 A2 L31 L52 L53 | L1 L2 L31 L45 L50 L53 | A2 L29 L30 L52 L53 | L35 L39 L40 A3 | L40 L42 A3 | L42 A3 L46 | L35 L39 L46 | L35 L39 A3 | L35 L39 A3 L46 | L38 L39 A3 L44 L59 | L42 A3 L44 L57 L58 L59 | L42 A3 L43 L51 | L36 L38 L39 A3 L59 bodies 1
sketch "Sketch6" plane through (0, 0, -19.2) normal (0, 0, -1) x (1, 0, 0)
  line L0 (19.4791, 229.1835) -> (22.8791, 225.7835)
  line L1 (22.8791, 225.1835) -> (98.0791, 225.1835)
  line L2 (98.0791, 225.7835) -> (101.4791, 229.1835)
  line L3 (101.4791, 229.1835) -> (113.0791, 229.1835)
  arc A0 (116.4791, 225.7835) -> (113.0791, 229.1835) centre (113.0791, 225.7835) ccw
  line L4 (116.4791, 225.7835) -> (116.4791, 5.5465)
  line L5 (116.4791, 5.5465) -> (113.0791, 3.5835)
  line L6 (113.0791, 3.5835) -> (113.0791, 219.1835)
  line L7 (111.4791, 219.1835) -> (111.4791, 5.1835)
  line L8 (111.4791, 5.1835) -> (9.4791, 5.1835)
  line L9 (9.4791, 5.1835) -> (9.4791, 219.1835)
  line L10 (7.8791, 219.1835) -> (7.8791, 3.5835)
  line L11 (7.8791, 3.5835) -> (4.4791, 5.5465)
  line L12 (4.4791, 5.5465) -> (4.4791, 225.7835)
  arc A1 (7.8791, 229.1835) -> (4.4791, 225.7835) centre (7.8791, 225.7835) ccw
  line L13 (7.8791, 229.1835) -> (19.4791, 229.1835)
  line L14 (2.0791, -2.2165) -> (118.8791, -2.2165)
  line L15 (118.8791, -2.2165) -> (118.8791, 232.5835)
  line L16 (118.8791, 232.5835) -> (2.0791, 232.5835)
  line L17 (2.0791, 232.5835) -> (2.0791, -2.2165)
  line L18 (9.4791, 5.1835) -> (9.4791, 225.1835)
  line L19 (111.4791, 5.1835) -> (9.4791, 5.1835)
  line L20 (111.4791, 225.1835) -> (111.4791, 5.1835)
  line L21 (9.4791, 225.1835) -> (111.4791, 225.1835)
  line L22 (2.0791, -2.2165) -> (2.0791, 232.5835)
  line L23 (2.0791, 232.5835) -> (118.8791, 232.5835)
  line L24 (118.8791, -2.2165) -> (2.0791, -2.2165)
  line L25 (118.8791, 232.5835) -> (118.8791, -2.2165)
  line L26 (29.4791, 229.3835) -> (91.4791, 229.3835)
  line L27 (91.4791, 229.3835) -> (91.4791, 228.3835)
  line L28 (91.4791, 228.3835) -> (29.4791, 228.3835)
  line L29 (29.4791, 228.3835) -> (29.4791, 229.3835)
  line L30 (28.0641, 232.5835) -> (28.0641, 225.1835) construction
  line L31 (28.0641, 229.3835) -> (28.0641, 228.3835) construction
  line L32 (111.4791, 115.1835) -> (9.4791, 115.1835)
  line L33 (29.4791, 0.9835) -> (108.4791, 0.9835)
  line L34 (108.4791, 1.9835) -> (29.4791, 1.9835)
  line L35 (29.4791, 1.9835) -> (29.4791, 0.9835)
  line L36 (91.4791, 0.9835) -> (91.4791, 1.9835)
  line L37 (29.0791, 229.7835) -> (91.8791, 229.7835)
  line L38 (91.8791, 229.7835) -> (91.8791, 227.9835)
  line L39 (91.8791, 227.9835) -> (29.0791, 227.9835)
  line L40 (29.0791, 227.9835) -> (29.0791, 229.7835)
  line L41 (91.8791, 2.3835) -> (29.0791, 2.3835)
  line L42 (29.0791, 0.5835) -> (91.8791, 0.5835)
  line L43 (29.0791, 2.3835) -> (29.0791, 0.5835)
  line L44 (60.4791, -3.0477) -> (60.4791, 233.4147)
  line L45 (42.4791, 227.9835) -> (42.4791, 229.7835)
  line L46 (78.4791, 227.9835) -> (78.4791, 229.7835)
  line L47 (42.8791, 227.9835) -> (42.8791, 229.7835)
  line L48 (78.0791, 227.9835) -> (78.0791, 229.7835)
  line L49 (39.0791, 2.3835) -> (108.4791, 2.3835)
  line L50 (108.4791, 2.3835) -> (108.4791, 0.5835)
  line L51 (108.4791, 0.5835) -> (39.0791, 0.5835)
  line L52 (39.0791, 0.5835) -> (39.0791, 2.3835)
  line L53 (88.4791, 2.3835) -> (88.4791, 0.5835)
  line L54 (39.4791, 2.3835) -> (39.4791, 0.5835)
  line L55 (22.8791, 225.7835) -> (22.8791, 225.1835)
  line L56 (98.0791, 225.1835) -> (98.0791, 225.7835)
  line L57 (113.0791, 219.1835) -> (111.4791, 219.1835)
  line L58 (9.4791, 219.1835) -> (7.8791, 219.1835)
  line L59 (88.0791, 2.3835) -> (88.0791, 0.5835)
  point P0 (28.0641, 228.8835)
  point P1 (28.0641, 228.8835)
  dimension "d120" = 10
  dimension "d121" = 10
  dimension "d122" = 1
  dimension "d123" = -0.4
  dimension "d147" = 18
  dimension "d148" = 18
  dimension "d149" = 0.4
  dimension "d150" = -0.4
  dimension "d153" = 1.8
  dimension "d154" = 10
  dimension "d155" = 3
  dimension "d156" = 20
  dimension "d158" = 90
  dimension "d159" = 0.4
  dimension "d196" = 0.4
  constraint horizontal L26
  constraint vertical L27
  constraint horizontal L28
  constraint vertical L29
  constraint coincident L16 L30.start
  constraint coincident L1 L30.end
  constraint perpendicular L1 L30
  constraint coincident L26 L31.start
  constraint coincident L28 L31.end
  constraint perpendicular L28 L31
  constraint midpoint L31 P1
  constraint midpoint L30 P1
  constraint coincident P1 P0
  constraint symmetric L26.start L32 L33.start
  constraint symmetric L26.end L32 L36.start
  constraint symmetric L27.end L32 L36.end
  constraint symmetric L28.end L32 L34.end
  constraint symmetric L32 L37.start L42.start
  constraint symmetric L32 L37.end L42.end
  constraint symmetric L32 L38.end L41.start
  constraint symmetric L32 L39.end L41.end
  constraint coincident L39 L45.start
  constraint coincident L37 L45.end
  constraint perpendicular L37 L45
  constraint coincident L39 L46.start
  constraint coincident L37 L46.end
  constraint perpendicular L37 L46
  constraint horizontal L49
  constraint vertical L50
  constraint horizontal L51
  constraint vertical L52
  constraint coincident L41 L49.start
  constraint coincident L36.end L34
  constraint coincident L50 L34.start
  constraint coincident L36.start L33
  constraint coincident L50 L33.end
  constraint coincident L49 L53.start
  constraint coincident L51 L53.end
  constraint perpendicular L51 L53
  constraint coincident L49 L54.start
  constraint coincident L42 L54.end
  constraint coincident L49 L59.start
  constraint coincident L51 L59.end
  constraint perpendicular L51 L59
  measures "d120" distance of L2.end L27
  measures "d121" distance of L0.start L29
  measures "d122" distance of L26 L28
  measures "d147" distance of L44 L46
  measures "d148" distance of L44 L45
  measures "d153" distance of L49 L51
  measures "d154" distance of L43 L52
  measures "d155" distance of L20 L50
  measures "d156" distance of L50 L53
  measures "d158" angle of L41 L54
  measures "d159" distance of L52 L54
  measures "d196" distance of L53 L59
extrude "Extrude9" add sketch "Sketch6" along normal blind 4.2 separate body contours L0 L1 L8 L9 L10 L11 L12 A1 L13 L14 L16 L17 L18 L19 L21 L22 L23 L24 L37 L39 L40 L41 L42 L43 L44 L49 L51 L55 L58 | L0 L10 L11 L12 A1 L13 L18 L21 L55 L58 | L1 L2 L3 A0 L4 L5 L6 L7 L8 L14 L15 L16 L19 L20 L21 L23 L24 L25 L37 L38 L39 L41 L42 L44 L49 L50 L51 L56 L57 | L2 L3 A0 L4 L5 L6 L20 L21 L56 L57 | L28 L39 L44 L48 | L28 L39 L44 L47 | L28 L39 L46 L48 | L28 L39 L45 L47 | L26 L28 L44 L48 | L26 L28 L44 L47 | L34 L41 L44 L49 L54 | L34 L41 L44 L49 L59 | L26 L27 L28 L37 L38 L39 L46 | L26 L28 L46 L48 | L26 L28 L29 L37 L39 L40 L45 | L26 L28 L45 L47 | L26 L37 L44 L48 | L26 L37 L44 L47 | L34 L41 L49 L53 L59 | L34 L41 L49 L52 L54 | L33 L34 L44 L54 | L33 L34 L44 L59 | L26 L27 L28 L46 | L26 L37 L46 L48 | L26 L28 L29 L45 | L26 L37 L45 L47 | L34 L41 L49 L50 L53 | L33 L34 L53 L59 | L33 L34 L35 L41 L42 L43 L52 | L33 L34 L52 L54 | L33 L42 L44 L51 L54 | L33 L42 L44 L51 L59 | L33 L34 L36 L53 | L33 L42 L51 L53 L59 | L33 L34 L35 L52 | L33 L42 L51 L52 L54 | L33 L34 L36 L50 | L33 L42 L50 L51 L53 makes body 2
sketch "Sketch7" plane through (0, 0, -23.4) normal (0, 0, -1) x (1, 0, 0)
  line L0 (9.4791, 5.1835) -> (9.4791, 225.1835)
  line L1 (9.4791, 225.1835) -> (111.4791, 225.1835)
  line L2 (111.4791, 225.1835) -> (111.4791, 5.1835)
  line L3 (111.4791, 5.1835) -> (9.4791, 5.1835)
  line L4 (118.8791, 232.5835) -> (2.0791, 232.5835)
  line L5 (2.0791, 232.5835) -> (2.0791, -2.2165)
  line L6 (2.0791, -2.2165) -> (118.8791, -2.2165)
  line L7 (118.8791, -2.2165) -> (118.8791, 232.5835)
  circle A0 centre (107.1093, 9.6234) radius 1.85
  circle A1 centre (13.8605, 9.6234) radius 1.85
  circle A2 centre (13.8605, 220.7337) radius 1.85
  circle A3 centre (107.1093, 220.7337) radius 1.85
  circle A4 centre (106.1086, 111.1767) radius 1.85
  circle A5 centre (13.8605, 111.1767) radius 1.85
extrude "Extrude10" add sketch "Sketch7" along normal blind 1.8 contours L0 L1 L2 L3 | L4 L5 L6 L7 bodies 2
extrude "Extrude11" cut sketch "Sketch6" along normal blind 2 contours L28 L39 L46 L48 | L28 L39 L45 L47 | L34 L41 L44 L49 L54 | L34 L41 L44 L49 L59 | L26 L27 L28 L37 L38 L39 L46 | L26 L28 L46 L48 | L26 L28 L29 L37 L39 L40 L45 | L26 L28 L45 L47 | L34 L41 L49 L53 L59 | L34 L41 L49 L52 L54 | L33 L34 L44 L54 | L33 L34 L44 L59 | L26 L27 L28 L46 | L26 L37 L46 L48 | L26 L28 L29 L45 | L26 L37 L45 L47 | L33 L34 L53 L59 | L33 L34 L52 L54 | L33 L42 L44 L51 L54 | L33 L42 L44 L51 L59 | L33 L42 L51 L53 L59 | L33 L42 L51 L52 L54 bodies 2
extrude "Extrude12" add sketch "Sketch6" along normal blind 1.6 contours L33 L34 L44 L54 | L33 L34 L44 L59 | L26 L27 L28 L46 | L26 L28 L29 L45 bodies 1